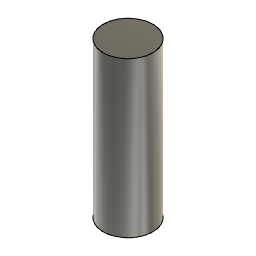
Lymphedema Project  Assembly v59 (Autodesk Fusion 360 archive; units mm, degrees)
design "Hand Model"
Autodesk Fusion 360 part; units mm, degrees
note: some values were not read from the file. Chosen so that the rebuilt part matches the saved one: that a step has no effect; which face or edge a step refers to. Set by a fixed rule: which sketch regions a step uses.
sketch "Sketch1" plane through (0, 0, 0) normal (0, 1, 0) x (1, 0, 0)
  circle A0 through (40, 0, 0) (-20, 0, 34.641) (-20, 0, -34.641)
  dimension "d1" = 80
sketch "Sketch1 (curves on the plane with normal 0, 0, -1 at 0 mm)" plane through (0, 0, 0) normal (0, 0, -1) x (-1, 0, 0)
  circle A0 centre (0, 0) radius 40
extrude "Extrude1" add sketch "Sketch1 (curves on the plane with normal 0, 0, -1 at 0 mm)" against normal blind 250

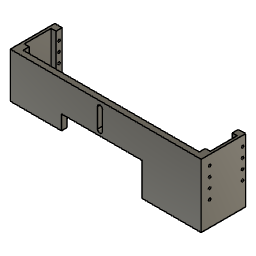
design "Motor case 2"
Autodesk Fusion 360 part; units mm, degrees
sketch "Sketch1" plane through (0, 0, 0) normal (0, 0, 1) x (1, 0, 0)
  line L0 (0, 0) -> (144.5, 0)
  line L1 (0, 0) -> (0, 5)
  line L2 (144.5, 0) -> (144.5, 5)
  line L3 (0, 5) -> (-4, 5)
  line L4 (144.5, 5) -> (148.5, 5)
  line L5 (-4, 5) -> (-4, 27)
  line L6 (-4, 27) -> (0, 27)
  line L7 (0, 27) -> (0, 32)
  line L8 (148.5, 5) -> (148.5, 27)
  line L9 (148.5, 27) -> (144.5, 27)
  line L10 (144.5, 27) -> (144.5, 32)
  line L11 (0, 32) -> (-6, 32)
  line L12 (-6, 32) -> (-6, -3)
  line L13 (-6, -3) -> (150.5, -3)
  line L14 (150.5, -3) -> (150.5, 32)
  line L15 (150.5, 32) -> (144.5, 32)
  dimension "d2" = 5
  dimension "d3" = 5
  dimension "d4" = 4
  dimension "d5" = 4
  dimension "d6" = 22
  dimension "d7" = 22
  dimension "d8" = 5
  dimension "d10" = 6
  dimension "d11" = 35
  dimension "d12" = 156.5
  dimension "d13" = 35
  dimension "d83" = 2
  dimension "d84" = 2
  dimension "d85" = 6
  dimension "d86" = 6
  dimension "d87" = 6
  constraint coincident L0.start L1.start
  constraint horizontal L0
  constraint perpendicular L0 L1
  constraint perpendicular L0 L2
  constraint perpendicular L1 L3
  constraint perpendicular L2 L4
  constraint perpendicular L3 L5
  constraint perpendicular L5 L6
  constraint perpendicular L6 L7
  constraint perpendicular L4 L8
  constraint perpendicular L8 L9
  constraint perpendicular L9 L10
  constraint perpendicular L7 L11
  constraint perpendicular L11 L12
  constraint perpendicular L12 L13
  constraint perpendicular L13 L14
  measures "d2" distance of L0.start L1.end
  measures "d3" distance of L0.end L2.end
  measures "d4" distance of L1.end L3.end
  measures "d5" distance of L2.end L4.end
  measures "d6" distance of L3.end L5.end
  measures "d7" distance of L4.end L8.end
  measures "d8" distance of L9.end L10.end
  measures "d10" distance of L7.end L11.end
  measures "d11" distance of L11.end L12.end
  measures "d12" distance of L12.end L13.end
  measures "d13" distance of L13.end L14.end
  measures "d83" distance of L8 L14
  measures "d84" distance of L5 L12
  measures "d85" distance of L10 L14
  measures "d86" distance of L2 L14
  measures "d87" distance of L1 L12
extrude "Extrude1" add sketch "Sketch1" along normal blind 37
sketch "Sketch2" plane through (-6, 0, 0) normal (-1, 0, 0) x (0, -1, 0)
  line L0 (-32, 0) -> (3, 0)
  line L1 (3, 0) -> (3, 37)
  line L2 (3, 37) -> (-32, 37)
  line L3 (-32, 37) -> (-32, 0)
  line L4 (-27, 37) -> (-32, 37)
  circle A0 centre (-29.5, 5) radius 1
  circle A1 centre (-29.5, 13) radius 1
  circle A2 centre (-29.5, 21) radius 1
  circle A3 centre (-29.5, 29) radius 1
  circle A4 centre (-2.5, 29) radius 1
  circle A5 centre (-2.5, 21) radius 1
  circle A6 centre (-2.5, 13) radius 1
  circle A7 centre (-2.5, 5) radius 1
  dimension "d18" = 2
  dimension "d19" = 2
  dimension "d21" = 2
  dimension "d22" = 8
  dimension "d24" = 8
  dimension "d25" = 2
  dimension "d26" = 8
  measures "d18" diameter of A0
  measures "d19" diameter of A1
  measures "d21" diameter of A2
  measures "d22" distance of A0.centre A1.centre
  measures "d24" distance of A1.centre A2.centre
  measures "d25" diameter of A3
  measures "d26" distance of A2.centre A3.centre
hole "Hole2" at (-6, 2.5, 29) at (-6, 2.5, 21) at (-6, 2.5, 13) at (-6, 2.5, 5) direction (1, 0, 0) diameter 2 depth 80 tip angle 118
hole "Hole3" at (-6, 29.5, 29) direction (1, 0, 0) diameter 2 depth 280 tip angle 118
hole "Hole4" at (-6, 29.5, 21) at (-6, 29.5, 13) at (-6, 29.5, 5) at (-6, 2.5, 29) at (-6, 2.5, 21) at (-6, 2.5, 13) at (-6, 2.5, 5) direction (1, 0, 0) diameter 2 depth 245 tip angle 118
sketch "Sketch3" plane through (0, -3, 0) normal (0, -1, 0) x (1, 0, 0)
  line L0 (-6, 0) -> (150.5, 0)
  line L1 (150.5, 0) -> (150.5, 37)
  line L2 (150.5, 37) -> (-6, 37)
  line L3 (-6, 37) -> (-6, 0)
  line L4 (36, 0) -> (36, 12)
  line L5 (36, 12) -> (102, 12)
  line L6 (102, 12) -> (102, 0)
  line L7 (36, 0) -> (102, 0)
  line L8 (-6, 0) -> (-6, 37)
  dimension "d45" = 12
  dimension "d79" = 12
  dimension "d81" = 42
  dimension "d82" = 66
  constraint coincident L0 L6.end
  constraint perpendicular L0 L4
  constraint perpendicular L4 L5
  constraint perpendicular L0 L6
  constraint perpendicular L6 L7
  measures "d45" distance of L4.start L4.end
  measures "d79" distance of L6.end L5.end
  measures "d81" distance of L4 L8
  measures "d82" distance of L4.end L5.end
extrude "Extrude2" cut sketch "Sketch3" against normal blind 9 contours L0 L4 L5 L6 L7
sketch "Sketch4" plane through (150.5, 0, 0) normal (1, 0, 0) x (0, 1, 0)
  line L0 (-3, 0) -> (32, 0)
  line L1 (32, 0) -> (32, 37)
  line L2 (32, 37) -> (-3, 37)
  line L3 (-3, 37) -> (-3, 0)
  circle A0 centre (14.5, 44) radius 2.1
  line L4 (14.5, 49.1) -> (10, 49.1)
  line L5 (10, 49.1) -> (10, 37)
  line L6 (19, 49.1) -> (19, 37)
  line L7 (19, 37) -> (14.5, 37)
  line L8 (19, 49.1) -> (14.5, 49.1)
  circle A1 centre (2.5, 13) radius 1
  circle A2 centre (2.5, 29) radius 1
  circle A3 centre (29.5, 13) radius 1
  circle A4 centre (29.5, 21) radius 1
  circle A5 centre (29.5, 5) radius 1
  circle A6 centre (2.5, 21) radius 1
  circle A7 centre (2.5, 5) radius 1
  circle A8 centre (29.5, 29) radius 1
  dimension "d46" = 17.5
  dimension "d47" = 7
  dimension "d48" = 4.2
  measures "d46" distance of L2.end L7.end
  measures "d47" distance of L7.end A0.centre
  measures "d48" diameter of A0
sketch "Sketch5" plane through (150.5, 0, 0) normal (1, 0, 0) x (0, 1, 0)
  line L0 (32, 37) -> (-3, 37)
  line L1 (-3, 37) -> (-3, 0)
  line L2 (-3, 0) -> (32, 0)
  line L3 (32, 0) -> (32, 37)
  line L4 (6.9, 0) -> (6.9, 10)
  line L5 (22.1, 0) -> (22.1, 37)
  line L6 (22.1, 0) -> (24.1, 0)
  line L7 (24.1, 0) -> (24.1, 37)
  line L8 (6.9, 0) -> (4.9, 0)
  line L9 (4.9, 0) -> (4.927, 10.0053)
  line L10 (6.9, 0) -> (6.9, 10)
  line L11 (6.9, 10) -> (4.9, 10.0054)
  circle A0 centre (2.5, 13) radius 1
  circle A1 centre (2.5, 29) radius 1
  circle A2 centre (29.5, 13) radius 1
  circle A3 centre (29.5, 21) radius 1
  circle A4 centre (29.5, 5) radius 1
  circle A5 centre (2.5, 21) radius 1
  circle A6 centre (2.5, 5) radius 1
  circle A7 centre (29.5, 29) radius 1
  point P0 (5, 37)
  point P1 (5, 37)
  dimension "d54" = 9.9
  dimension "d55" = 9.9
  dimension "d56" = 2
  dimension "d57" = 2
  dimension "d60" = 10
  dimension "d61" = 2
  constraint coincident L2 L4.start
  constraint perpendicular L0 L4
  constraint perpendicular L5 L6
  constraint perpendicular L4 L8
  constraint perpendicular L2 L10
  constraint perpendicular L9 L11
  constraint coincident L11 L9.end
  measures "d54" distance of L1.end L4.start
  measures "d55" distance of L2.end L5.start
  measures "d56" distance of L5.start L6.end
  measures "d57" distance of L4.start L8.end
  measures "d60" distance of L4.start L4.end
  measures "d61" distance of L4.end L11.end
ref_plane "WorkPlane1" through (102.5, 14.5, 18.5) normal (1, 0, 0) x (0, 1, 0)
sketch "Sketch7" plane through (0, -3, 0) normal (0, -1, 0) x (1, 0, 0)
  line L0 (36, 0) -> (36, 12)
  line L1 (36, 12) -> (102, 12)
  line L2 (102, 12) -> (102, 0)
  line L3 (102, 0) -> (150.5, 0)
  line L4 (150.5, 0) -> (150.5, 37)
  line L5 (150.5, 37) -> (-6, 37)
  line L6 (-6, 37) -> (-6, 0)
  line L7 (-6, 0) -> (36, 0)
  line L8 (65.5, 32) -> (65.5, 16)
  line L9 (69.5, 32) -> (69.5, 16)
  arc A0 (69.5, 32) -> (65.5, 32) centre (67.5, 32) ccw
  arc A1 (65.5, 16) -> (69.5, 16) centre (67.5, 16) ccw
  dimension "d71" = 4
  dimension "d74" = 4
  dimension "d76" = 2
  dimension "d88" = 71.5
  dimension "d89" = 4
  constraint tangent L8 A0
  constraint perpendicular L1 L9
  measures "d71" diameter of A0
  measures "d74" distance of L8 L9
  measures "d76" radius of A0
  measures "d88" distance of L6 L8
  measures "d89" distance of L1 A1.centre
extrude "Extrude7" cut sketch "Sketch7" against normal blind 13 contours L8 L9 A0 A1
extrude "Extrude8" add 1 faces at (134.3333, -3, 16.3333) along direction (0, -1, 0) blind 1.5
extrude "Extrude9" add 1 faces at (132.3333, -3, 0) along direction (0, 0, -1) blind 15
sketch "Sketch8" plane through (0, 0, 0) normal (0, 1, 0) x (-1, 0, 0)
  line L0 (-65.5, 32) -> (-65.5, 16)
  arc A0 (-69.5, 16) -> (-65.5, 16) centre (-67.5, 16) ccw
  line L1 (-69.5, 16) -> (-69.5, 32)
  arc A1 (-65.5, 32) -> (-69.5, 32) centre (-67.5, 32) ccw
  line L2 (-36, 12) -> (-36, 0)
  line L3 (-36, 0) -> (0, 0)
  line L4 (0, 0) -> (0, 37)
  line L5 (0, 37) -> (-144.5, 37)
  line L6 (-144.5, 37) -> (-144.5, -15)
  line L7 (-144.5, -15) -> (-102, -15)
  line L8 (-102, -15) -> (-102, 12)
  line L9 (-102, 12) -> (-36, 12)
  line L10 (-102, 2.5) -> (-107, 2.5)
  line L11 (-102, -5.5) -> (-107, -5.5)
  line L12 (-107, -5.5) -> (-107, 2.5)
  line L13 (-102, 2.5) -> (-102, -5.5)
  dimension "d97" = 5
  dimension "d100" = 8
  dimension "d101" = 8
  dimension "d102" = 9.5
  constraint perpendicular L8 L10
  constraint perpendicular L8 L11
  constraint perpendicular L11 L13
  measures "d97" distance of L10.start L10.end
  measures "d100" distance of L10.end L11.end
  measures "d101" distance of L11.start L10.start
  measures "d102" distance of L7 L11
extrude "Extrude10" add sketch "Sketch8" along normal blind 25 contours L8 L10 L11 L12 L13
sketch "Sketch10" plane through (102, 0, 0) normal (-1, 0, 0) x (0, -1, 0)
  line L0 (0, -5.5) -> (0, -15)
  line L1 (0, -15) -> (4.5, -15)
  line L2 (4.5, -15) -> (4.5, 12)
  line L3 (4.5, 12) -> (0, 12)
  line L4 (0, 12) -> (0, 2.5)
  line L5 (0, 2.5) -> (-25, 2.5)
  line L6 (-25, 2.5) -> (-25, -5.5)
  line L7 (-25, -5.5) -> (0, -5.5)
  circle A0 centre (-16, -1.5) radius 2.5
  dimension "d107" = 5
  dimension "d108" = 9
  measures "d107" diameter of A0
  measures "d108" distance of L6 A0.centre
extrude "Extrude12" add sketch "Sketch10" along normal blind 6 contours A0
fillet "Fillet4" radius 2 1 edges at (96, 18.3308, -2.404)
fillet "Fillet5" radius 4 2 edges at (104.5, 0, -5.5) (104.5, 0, 2.5)
equation "d11 = 32.00 mm + 3 mm"
equation "d12 = 96 mm + 10.5 mm + 50 mm"
equation "d46 = ( 35 / 2 ) * 1 mm"
equation "d64 = ( -96 / 2 ) * 1 mm"
equation "d88 = 46.50 mm + 25 mm"

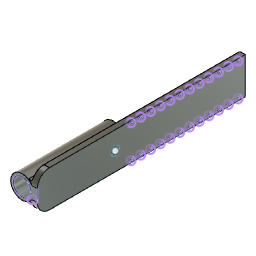
design "dummy wheel bracket"
Autodesk Fusion 360 part; units mm, degrees
sketch "Sketch1" plane through (0, 0, 0) normal (0, 0, 1) x (1, 0, 0)
  line L0 (-50.5, 0) -> (-50.5, -67)
  line L1 (-50.5, -67) -> (-55, -67)
  line L2 (-55, -67) -> (-55, 103.982)
  line L3 (-55, 103.982) -> (-50.5, 103.982)
  line L4 (-50.5, 0) -> (-50.5, 103.982)
  dimension "d3" = 4.5
  dimension "d42" = 170.982
  constraint perpendicular L0 L1
  constraint perpendicular L1 L2
  constraint perpendicular L2 L3
  constraint perpendicular L3 L4
  measures "d3" distance of L0.end L1.end
  measures "d42" distance of L1.end L2.end
extrude "Extrude1" add sketch "Sketch1" along normal blind 30
sketch "Sketch3" plane through (-50.5, 0, 0) normal (1, 0, 0) x (0, 1, 0)
  line L0 (-67, 0) -> (103.982, 0)
  line L1 (103.982, 30) -> (-67, 30)
  line L2 (-67, 30) -> (-67, 0)
  circle A0 centre (-62, 15) radius 2.1
  line L3 (103.982, 0) -> (103.982, 30)
  dimension "d14" = 4.2
  dimension "d17" = 5
  measures "d14" diameter of A0
  measures "d17" distance of L2 A0.centre
extrude "Extrude3" cut sketch "Sketch3" against normal blind 12 contours A0
sketch "Sketch4" plane through (-50.5, 0, 0) normal (1, 0, 0) x (0, 1, 0)
  circle A0 centre (-62, 15) radius 2.1
  line L0 (-67, 0) -> (103.982, 0)
  line L1 (103.982, 0) -> (103.982, 30)
  line L2 (103.982, 30) -> (-67, 30)
  line L3 (-67, 30) -> (-67, 0)
  line L4 (-67, 15) -> (-59.9, 15)
  circle A1 centre (57.982, 28.5) radius 1
  circle A2 centre (65.982, 28.5) radius 1
  circle A3 centre (81.982, 28.5) radius 1
  circle A4 centre (73.982, 28.5) radius 1
  circle A5 centre (65.982, 1.5) radius 1
  circle A6 centre (73.982, 1.5) radius 1
  circle A7 centre (81.982, 1.5) radius 1
  circle A8 centre (57.982, 1.5) radius 1
  circle A9 centre (89.982, 28.5) radius 1
  circle A10 centre (97.982, 28.5) radius 1
  circle A11 centre (89.982, 1.5) radius 1
  circle A12 centre (97.982, 1.5) radius 1
  circle A13 centre (49.982, 28.5) radius 1
  circle A14 centre (41.982, 28.5) radius 1
  circle A15 centre (33.982, 28.5) radius 1
  circle A16 centre (49.982, 1.5) radius 1
  circle A17 centre (41.982, 1.5) radius 1
  circle A18 centre (33.982, 1.5) radius 1
  circle A19 centre (25.982, 1.5) radius 1
  circle A20 centre (25.982, 28.5) radius 1
  circle A21 centre (17.982, 28.5) radius 1
  circle A22 centre (17.982, 1.5) radius 1
  circle A23 centre (9.982, 28.5) radius 1
  circle A24 centre (9.982, 1.5) radius 1
  dimension "d20" = 2
  dimension "d21" = 13.5
  dimension "d22" = 2
  dimension "d23" = 13.5
  dimension "d24" = 8
  dimension "d29" = 124.982
  dimension "d30" = 8
  dimension "d31" = 8
  dimension "d32" = 27
  dimension "d33" = 8
  dimension "d34" = 8
  dimension "d35" = 8
  dimension "d36" = 2
  dimension "d37" = 2
  dimension "d38" = 2
  dimension "d39" = 2
  dimension "d40" = 2
  dimension "d41" = 2
  constraint midpoint L3 L4.start
  constraint symmetric L4 A1 A8
  constraint symmetric L4 A2 A5
  constraint symmetric L4 A3 A7
  constraint symmetric L4 A4 A6
  constraint coincident A0 L4.end
  measures "d20" diameter of A1
  measures "d21" distance of L4 A1.centre
  measures "d22" diameter of A2
  measures "d23" distance of L4 A2.centre
  measures "d24" distance of A1.centre A2.centre
  measures "d29" distance of L3 A1.centre
  measures "d30" distance of A2.centre A4.centre
  measures "d31" distance of A3.centre A4.centre
  measures "d32" distance of A1.centre A8.centre
  measures "d33" distance of A5.centre A8.centre
  measures "d34" distance of A5.centre A6.centre
  measures "d35" distance of A6.centre A7.centre
  measures "d36" diameter of A3
  measures "d37" diameter of A4
  measures "d38" diameter of A7
  measures "d39" diameter of A6
  measures "d40" diameter of A5
  measures "d41" diameter of A8
hole "Hole1" at (-50.5, 9.982, 28.5) at (-50.5, 17.982, 28.5) at (-50.5, 25.982, 28.5) at (-50.5, 33.982, 28.5) at (-50.5, 41.982, 28.5) at (-50.5, 49.982, 28.5) at (-50.5, 57.982, 28.5) at (-50.5, 65.982, 28.5) at (-50.5, 73.982, 28.5) at (-50.5, 81.982, 28.5) at (-50.5, 89.982, 28.5) at (-50.5, 97.982, 28.5) at (-50.5, 97.982, 1.5) at (-50.5, 89.982, 1.5) at (-50.5, 81.982, 1.5) at (-50.5, 73.982, 1.5) at (-50.5, 65.982, 1.5) at (-50.5, 57.982, 1.5) at (-50.5, 49.982, 1.5) at (-50.5, 41.982, 1.5) at (-50.5, 33.982, 1.5) at (-50.5, 25.982, 1.5) at (-50.5, 17.982, 1.5) at (-50.5, 9.982, 1.5) direction (-1, 0, 0) diameter 2 depth 9 tip angle 118
fillet "Fillet3" radius 10 2 edges at (-52.75, -67, 30) (-52.75, -67, 0)
fillet "Fillet4" [no effect]
sketch "Sketch5" plane through (0, -67, 0) normal (0, -1, 0) x (1, 0, 0)
  line L0 (-55, 10) -> (-50.5, 10)
  line L1 (-50.5, 10) -> (-50.5, 20)
  line L2 (-50.5, 20) -> (-55, 20)
  line L3 (-55, 20) -> (-55, 10)
  line L4 (-55, 30) -> (-50.5, 30)
  line L5 (-50.5, 29.5) -> (-50.5, 27.5)
  line L6 (-50.5, 0) -> (-55, 0)
  circle A0 centre (-63, 15) radius 7.25
  line L7 (-55, 20) -> (-55, 10)
  arc A1 (-55, 20) -> (-55, 10) centre (-63, 15) ccw
  point P0 (-55, 30)
  dimension "d49" = 14.5
  dimension "d50" = 8
  constraint concentric A0 A1
  constraint coincident L2.end L3.start
  constraint coincident L0.start L3.end
  measures "d49" diameter of A0
  measures "d50" distance of L3 A0.centre
extrude "Extrude5" add sketch "Sketch5" against normal blind 70
sketch "Sketch6" plane through (0, -67, 0) normal (0, -1, 0) x (1, 0, 0)
  circle A0 centre (-63, 15) radius 7.25
  line L0 (-55, 10) -> (-50.5, 10)
  line L1 (-50.5, 20) -> (-55, 20)
  arc A1 (-55, 20) -> (-55, 10) centre (-63, 15) ccw
  circle A2 centre (-63, 15) radius 5
  circle A3 centre (-63, 15) radius 7
  line L2 (-50.5, 10) -> (-50.5, 20)
  dimension "d52" = 14
  constraint concentric A0 A2
  constraint concentric A2 A3
  measures "d52" diameter of A3
sketch "Sketch7" plane through (-50.5, 0, 0) normal (1, 0, 0) x (0, 1, 0)
  arc A0 (-67, 10) -> (-57, 0) centre (-57, 10) ccw
  line L0 (-57, 0) -> (103.982, 0)
  line L1 (103.982, 0) -> (103.982, 30)
  line L2 (103.982, 30) -> (-57, 30)
  arc A1 (-57, 30) -> (-67, 20) centre (-57, 20) ccw
  circle A2 centre (-3, 15) radius 3
  line L3 (-67, 20) -> (-67, 10)
  circle A3 centre (41.982, 28.5) radius 1
  circle A4 centre (25.982, 28.5) radius 1
  circle A5 centre (9.982, 28.5) radius 1
  circle A6 centre (17.982, 28.5) radius 1
  circle A7 centre (33.982, 28.5) radius 1
  circle A8 centre (9.982, 1.5) radius 1
  circle A9 centre (25.982, 1.5) radius 1
  circle A10 centre (41.982, 1.5) radius 1
  circle A11 centre (57.982, 1.5) radius 1
  circle A12 centre (73.982, 1.5) radius 1
  circle A13 centre (89.982, 1.5) radius 1
  circle A14 centre (97.982, 28.5) radius 1
  circle A15 centre (81.982, 28.5) radius 1
  circle A16 centre (65.982, 28.5) radius 1
  circle A17 centre (49.982, 28.5) radius 1
  circle A18 centre (57.982, 28.5) radius 1
  circle A19 centre (73.982, 28.5) radius 1
  circle A20 centre (89.982, 28.5) radius 1
  circle A21 centre (97.982, 1.5) radius 1
  circle A22 centre (81.982, 1.5) radius 1
  circle A23 centre (65.982, 1.5) radius 1
  circle A24 centre (49.982, 1.5) radius 1
  circle A25 centre (33.982, 1.5) radius 1
  circle A26 centre (17.982, 1.5) radius 1
  dimension "d56" = 6
  dimension "d61" = 64
  measures "d56" diameter of A2
  measures "d61" distance of A2.centre L3
extrude "Extrude9" cut sketch "Sketch7" against normal blind 30 contours A2
sketch "Sketch9" plane through (0, -67, 0) normal (0, -1, 0) x (1, 0, 0)
  line L0 (-55, 10) -> (-50.5, 10)
  line L1 (-50.5, 10) -> (-50.5, 20)
  line L2 (-50.5, 20) -> (-55, 20)
  arc A0 (-55, 20) -> (-55, 10) centre (-63, 15) ccw
  circle A1 centre (-63, 15) radius 7.25
extrude "Extrude10" add 1 faces at (-71.6889, 3, 15) along direction (0, 1, 0) blind 5
fillet "Fillet7" radius 2 2 edges at (-55, -29.5, 10) (-55, -29.5, 20)
sketch "Sketch10" plane through (0, 8, 0) normal (0, 1, 0) x (-1, 0, 0)
  line L0 (55, 24.7332) -> (55, 5.2668)
  arc A0 (58.0495, 6.9693) -> (55, 5.2668) centre (57, 5.2668) ccw
  arc A1 (58.0495, 6.9693) -> (58.0495, 23.0307) centre (63, 15) ccw
  arc A2 (55, 24.7332) -> (58.0495, 23.0307) centre (57, 24.7332) ccw
  circle A3 centre (63, 15) radius 7.25
  circle A4 centre (63, 15) radius 7.25
  constraint concentric A1 A4
extrude "Extrude11" add sketch "Sketch10" against normal blind 2 contours A3 A4
equation "d21 = ( 27 / 2 ) * 1 mm"
equation "d29 = 45 mm + 31 mm + 48.982 mm"
equation "d42 = 72.00 mm + 50 mm + 48.982 mm"
